Autodesk Fusion 360 part; units mm, degrees
(part 4 of 5)
  spline S251 degree 3 poles (-20.8842, 19.6004) (-20.7556, 19.6004) (-20.6902, 19.4873) (-20.7714, 19.4061) knots 0 0 0 0 1 1 1 1
  spline S252 degree 3 poles (-20.7714, 19.4061) (-20.8663, 19.3108) (-21.0022, 19.3689) (-20.9874, 19.4986) knots 0 0 0 0 1 1 1 1
  spline S253 degree 3 poles (-20.9874, 19.4986) (-20.9781, 19.577) (-20.9547, 19.6004) (-20.8842, 19.6004) knots 0 0 0 0 1 1 1 1
  spline S254 degree 3 poles (-15.859, 20.19) (-15.7052, 20.0307) (-15.4972, 19.7727) (-15.3967, 19.6166) knots 0 0 0 0 1 1 1 1
  spline S255 degree 3 poles (-15.3967, 19.6166) (-15.0184, 19.0281) (-14.932, 18.9156) (-14.7484, 18.7698) knots 0 0 0 0 1 1 1 1
  spline S256 degree 3 poles (-14.7484, 18.7698) (-14.5557, 18.6167) (-14.2304, 18.4347) (-14.1499, 18.4347) knots 0 0 0 0 1 1 1 1
  spline S257 degree 3 poles (-14.1499, 18.4347) (-14.1251, 18.4347) (-14.2407, 18.5764) (-14.4068, 18.7501) knots 0 0 0 0 1 1 1 1
  spline S258 degree 3 poles (-14.4068, 18.7501) (-14.5726, 18.9235) (-14.7934, 19.2028) (-14.8973, 19.371) knots 0 0 0 0 1 1 1 1
  spline S259 degree 3 poles (-14.8973, 19.371) (-15.2719, 19.9774) (-15.5315, 20.2477) (-15.9388, 20.4548) knots 0 0 0 0 1 1 1 1
  spline S260 degree 3 poles (-15.9388, 20.4548) (-16.2274, 20.6013) (-16.214, 20.557) (-15.859, 20.19) knots 0 0 0 0 1 1 1 1
  spline S261 degree 3 poles (-15.6155, 21.0271) (-15.2839, 20.7069) (-14.9551, 20.5714) (-14.3803, 20.5181) knots 0 0 0 0 1 1 1 1
  spline S262 degree 3 poles (-14.3803, 20.5181) (-13.7203, 20.4569) (-12.3448, 20.6853) (-12.2268, 20.8755) knots 0 0 0 0 1 1 1 1
  spline S263 degree 3 poles (-12.2268, 20.8755) (-12.2185, 20.8889) (-12.7586, 20.894) (-13.4265, 20.8875) knots 0 0 0 0 1 1 1 1
  spline S264 degree 3 poles (-13.4265, 20.8875) (-14.7814, 20.8737) (-14.9286, 20.8889) (-15.3916, 21.0928) knots 0 0 0 0 1 1 1 1
  spline S265 degree 3 poles (-15.3916, 21.0928) (-15.5622, 21.1682) (-15.7231, 21.2387) (-15.7493, 21.2504) knots 0 0 0 0 1 1 1 1
  spline S266 degree 3 poles (-15.7493, 21.2504) (-15.849, 21.2934) (-15.7905, 21.1964) (-15.6155, 21.0271) knots 0 0 0 0 1 1 1 1
  spline S267 degree 3 poles (-13.7519, -14.1202) (-12.6942, -27.0541) (-11.8189, -37.6776) (-11.8061, -37.7278) knots 0 0 0 0 1 1 1 1
  spline S268 degree 3 poles (-11.8061, -37.7278) (-11.7607, -37.9101) (-11.4151, -37.9504) (-11.326, -37.7842) knots 0 0 0 0 1 1 1 1
  spline S269 degree 3 poles (-11.326, -37.7842) (-11.2393, -37.6222) (-11.2764, 12.0151) (-11.3638, 12.1578) knots 0 0 0 0 1 1 1 1
  spline S270 degree 3 poles (-11.3638, 12.1578) (-11.5103, 12.3983) (-11.8199, 12.5135) (-12.0768, 12.4234) knots 0 0 0 0 1 1 1 1
  spline S271 degree 3 poles (-12.0768, 12.4234) (-12.3517, 12.3267) (-15.5192, 10.2626) (-15.6048, 10.1244) knots 0 0 0 0 1 1 1 1
  spline S272 degree 3 poles (-15.6048, 10.1244) (-15.7235, 9.9324) (-15.7985, 10.9155) (-13.7519, -14.1202) knots 0 0 0 0 1 1 1 1
  spline S273 degree 3 poles (-15.6055, 47.6423) (-15.59, 47.5739) (-15.5364, 47.4665) (-15.4865, 47.4036) knots 0 0 0 0 1 1 1 1
  spline S274 degree 3 poles (-15.4865, 47.4036) (-15.3713, 47.2584) (-12.158, 45.1985) (-11.9657, 45.1462) knots 0 0 0 0 1 1 1 1
  spline S275 degree 3 poles (-11.9657, 45.1462) (-11.6961, 45.0736) (-11.3941, 45.2143) (-11.273, 45.4688) knots 0 0 0 0 1 1 1 1
  spline S276 degree 3 poles (-11.273, 45.4688) (-11.2159, 45.5896) (-11.2111, 47.5797) (-11.2111, 70.4615) knots 0 0 0 0 1 1 1 1
  line L116 (-11.2111, 70.4615) -> (-11.2111, 95.3228)
  line L117 (-11.2111, 95.3228) -> (-11.3115, 95.4023)
  spline S277 degree 3 poles (-11.3115, 95.4023) (-11.4347, 95.4989) (-11.5578, 95.5031) (-11.6675, 95.4143) knots 0 0 0 0 1 1 1 1
  spline S278 degree 3 poles (-11.6675, 95.4143) (-11.748, 95.349) (-11.7989, 94.7477) (-13.6755, 71.729) knots 0 0 0 0 1 1 1 1
  spline S279 degree 3 poles (-13.6755, 71.729) (-14.7346, 58.7391) (-15.6082, 48.0334) (-15.6172, 47.9388) knots 0 0 0 0 1 1 1 1
  spline S280 degree 3 poles (-15.6172, 47.9388) (-15.6261, 47.8442) (-15.6206, 47.7108) (-15.6055, 47.6423) knots 0 0 0 0 1 1 1 1
  spline S281 degree 3 poles (-15.1442, 24.6133) (-14.6259, 24.1441) (-13.8018, 23.8731) (-13.1434, 23.9553) knots 0 0 0 0 1 1 1 1
  spline S282 degree 3 poles (-13.1434, 23.9553) (-12.8686, 23.9897) (-12.8755, 24.0144) (-13.1888, 24.1235) knots 0 0 0 0 1 1 1 1
  spline S283 degree 3 poles (-13.1888, 24.1235) (-13.4503, 24.2146) (-15.2412, 24.8506) (-15.329, 24.8836) knots 0 0 0 0 1 1 1 1
  spline S284 degree 3 poles (-15.329, 24.8836) (-15.4404, 24.9256) (-15.3609, 24.809) (-15.1442, 24.6133) knots 0 0 0 0 1 1 1 1
  spline S285 degree 3 poles (-10.2752, 18.574) (-10.171, 18.9245) (-9.569, 19.6589) (-9.3878, 19.6568) knots 0 0 0 0 1 1 1 1
  spline S286 degree 3 poles (-9.3878, 19.6568) (-9.0524, 19.6527) (-8.8275, 19.3913) (-8.8797, 19.0659) knots 0 0 0 0 1 1 1 1
  spline S287 degree 3 poles (-8.8797, 19.0659) (-8.9637, 18.5403) (-9.1202, 18.3512) (-9.5436, 18.2624) knots 0 0 0 0 1 1 1 1
  spline S288 degree 3 poles (-9.5436, 18.2624) (-9.686, 18.2325) (-9.8573, 18.1744) (-9.9243, 18.1327) knots 0 0 0 0 1 1 1 1
  spline S289 degree 3 poles (-9.9243, 18.1327) (-10.3061, 17.8968) (-10.43, 18.0523) (-10.2752, 18.574) knots 0 0 0 0 1 1 1 1
  spline S290 degree 3 poles (-4.9222, -19.0378) (-4.4427, -21.601) (-2.4986, -23.2055) (0.1206, -23.1997) knots 0 0 0 0 1 1 1 1
  spline S291 degree 3 poles (0.1206, -23.1997) (3.6706, -23.1918) (5.9848, -19.9675) (4.9739, -16.4378) knots 0 0 0 0 1 1 1 1
  spline S292 degree 3 poles (4.9739, -16.4378) (3.682, -11.9251) (-2.9984, -11.6857) (-4.6573, -16.0925) knots 0 0 0 0 1 1 1 1
  spline S293 degree 3 poles (-4.6573, -16.0925) (-4.9524, -16.8767) (-5.0738, -18.2264) (-4.9222, -19.0378) knots 0 0 0 0 1 1 1 1
  spline S294 degree 3 poles (-4.9242, 2.0967) (-4.4138, -0.7987) (-1.6762, -2.6382) (1.1996, -2.0184) knots 0 0 0 0 1 1 1 1
  spline S295 degree 3 poles (1.1996, -2.0184) (5.118, -1.174) (6.5392, 3.6521) (3.7927, 6.788) knots 0 0 0 0 1 1 1 1
  spline S296 degree 3 poles (3.7927, 6.788) (3.6317, 6.972) (3.479, 7.1223) (3.4529, 7.1223) knots 0 0 0 0 1 1 1 1
  spline S297 degree 3 poles (3.4529, 7.1223) (3.4102, 7.1223) (3.1217, 6.8375) (2.2081, 5.8937) knots 0 0 0 0 1 1 1 1
  line L118 (2.2081, 5.8937) -> (1.8882, 5.5635)
  line L119 (1.8882, 5.5635) -> (2.0781, 5.3351)
  spline S298 degree 3 poles (2.0781, 5.3351) (3.8804, 3.1695) (2.7553, 0.3099) (0.1014, 0.3099) knots 0 0 0 0 1 1 1 1
  spline S299 degree 3 poles (0.1014, 0.3099) (-2.5523, 0.3099) (-3.6774, 3.1695) (-1.8757, 5.3344) knots 0 0 0 0 1 1 1 1
  line L120 (-1.8757, 5.3344) -> (-1.6865, 5.5621)
  line L121 (-1.6865, 5.5621) -> (-1.798, 5.6828)
  spline S300 degree 3 poles (-1.798, 5.6828) (-1.8592, 5.7496) (-2.2094, 6.1197) (-2.576, 6.5056) knots 0 0 0 0 1 1 1 1
  line L122 (-2.576, 6.5056) -> (-3.2426, 7.2076)
  line L123 (-3.2426, 7.2076) -> (-3.537, 6.8939)
  spline S301 degree 3 poles (-3.537, 6.8939) (-4.1995, 6.1881) (-4.6312, 5.387) (-4.8554, 4.447) knots 0 0 0 0 1 1 1 1
  spline S302 degree 3 poles (-4.8554, 4.447) (-4.9762, 3.94) (-5.0154, 2.6123) (-4.9242, 2.0967) knots 0 0 0 0 1 1 1 1
  spline S303 degree 3 poles (-4.9222, 21.5111) (-4.4427, 18.9479) (-2.4986, 17.3434) (0.1206, 17.3492) knots 0 0 0 0 1 1 1 1
  spline S304 degree 3 poles (0.1206, 17.3492) (3.6706, 17.3571) (5.9848, 20.5814) (4.9739, 24.1111) knots 0 0 0 0 1 1 1 1
  spline S305 degree 3 poles (4.9739, 24.1111) (3.682, 28.6238) (-2.9984, 28.8629) (-4.6573, 24.4561) knots 0 0 0 0 1 1 1 1
  spline S306 degree 3 poles (-4.6573, 24.4561) (-4.9524, 23.6722) (-5.0738, 22.3225) (-4.9222, 21.5111) knots 0 0 0 0 1 1 1 1
  spline S307 degree 3 poles (-4.9222, 44.3654) (-4.4427, 41.8022) (-2.4986, 40.1973) (0.1206, 40.2032) knots 0 0 0 0 1 1 1 1
  spline S308 degree 3 poles (0.1206, 40.2032) (3.6706, 40.2111) (5.9848, 43.4354) (4.9739, 46.9654) knots 0 0 0 0 1 1 1 1
  spline S309 degree 3 poles (4.9739, 46.9654) (3.682, 51.4778) (-2.9984, 51.7172) (-4.6573, 47.3104) knots 0 0 0 0 1 1 1 1
  spline S310 degree 3 poles (-4.6573, 47.3104) (-4.9524, 46.5262) (-5.0738, 45.1765) (-4.9222, 44.3654) knots 0 0 0 0 1 1 1 1
  spline S311 degree 3 poles (-4.9222, 63.474) (-4.4427, 60.9108) (-2.4986, 59.3063) (0.1206, 59.3121) knots 0 0 0 0 1 1 1 1
  spline S312 degree 3 poles (0.1206, 59.3121) (3.6706, 59.32) (5.9848, 62.5443) (4.9739, 66.074) knots 0 0 0 0 1 1 1 1
  spline S313 degree 3 poles (4.9739, 66.074) (3.682, 70.5867) (-2.9984, 70.8258) (-4.6573, 66.419) knots 0 0 0 0 1 1 1 1
  spline S314 degree 3 poles (-4.6573, 66.419) (-4.9524, 65.6351) (-5.0738, 64.2854) (-4.9222, 63.474) knots 0 0 0 0 1 1 1 1
  spline S315 degree 3 poles (-4.9242, 84.6085) (-4.4138, 81.7131) (-1.6762, 79.8736) (1.1996, 80.4934) knots 0 0 0 0 1 1 1 1
  spline S316 degree 3 poles (1.1996, 80.4934) (5.118, 81.3378) (6.5392, 86.1639) (3.7927, 89.2998) knots 0 0 0 0 1 1 1 1
  spline S317 degree 3 poles (3.7927, 89.2998) (3.6317, 89.4835) (3.479, 89.6341) (3.4529, 89.6341) knots 0 0 0 0 1 1 1 1
  spline S318 degree 3 poles (3.4529, 89.6341) (3.4102, 89.6341) (3.1217, 89.3493) (2.2081, 88.4055) knots 0 0 0 0 1 1 1 1
  line L124 (2.2081, 88.4055) -> (1.8882, 88.0753)
  line L125 (1.8882, 88.0753) -> (2.0781, 87.8469)
  spline S319 degree 3 poles (2.0781, 87.8469) (3.8804, 85.6813) (2.7553, 82.8217) (0.1014, 82.8217) knots 0 0 0 0 1 1 1 1
  spline S320 degree 3 poles (0.1014, 82.8217) (-2.5523, 82.8217) (-3.6774, 85.6813) (-1.8757, 87.8462) knots 0 0 0 0 1 1 1 1
  line L126 (-1.8757, 87.8462) -> (-1.6865, 88.0739)
  line L127 (-1.6865, 88.0739) -> (-1.798, 88.1947)
  spline S321 degree 3 poles (-1.798, 88.1947) (-1.8592, 88.261) (-2.2094, 88.6315) (-2.576, 89.0174) knots 0 0 0 0 1 1 1 1
  line L128 (-2.576, 89.0174) -> (-3.2426, 89.7194)
  line L129 (-3.2426, 89.7194) -> (-3.537, 89.4057)
  spline S322 degree 3 poles (-3.537, 89.4057) (-4.1995, 88.6999) (-4.6312, 87.8988) (-4.8554, 86.9588) knots 0 0 0 0 1 1 1 1
  spline S323 degree 3 poles (-4.8554, 86.9588) (-4.9762, 86.4518) (-5.0154, 85.1241) (-4.9242, 84.6085) knots 0 0 0 0 1 1 1 1
  spline S324 degree 3 poles (-4.9252, 92.6341) (-4.5713, 91.0117) (-3.1164, 89.9402) (-1.5187, 90.126) knots 0 0 0 0 1 1 1 1
  spline S325 degree 3 poles (-1.5187, 90.126) (-0.1704, 90.2828) (0.499, 90.9728) (1.1549, 92.8828) knots 0 0 0 0 1 1 1 1
  spline S326 degree 3 poles (1.1549, 92.8828) (1.6144, 94.2208) (1.9742, 94.5482) (2.6239, 94.2194) knots 0 0 0 0 1 1 1 1
  spline S327 degree 3 poles (2.6239, 94.2194) (3.3851, 93.8342) (3.0343, 92.424) (2.1768, 92.424) knots 0 0 0 0 1 1 1 1
  line L130 (2.1768, 92.424) -> (2.0506, 92.424)
  line L131 (2.0506, 92.424) -> (2.0506, 91.2545)
  line L132 (2.0506, 91.2545) -> (2.0506, 90.085)
  line L133 (2.0506, 90.085) -> (2.3275, 90.1108)
  spline S328 degree 3 poles (2.3275, 90.1108) (4.2423, 90.2897) (5.3419, 91.6934) (5.1765, 93.7479) knots 0 0 0 0 1 1 1 1
  spline S329 degree 3 poles (5.1765, 93.7479) (4.9292, 96.8191) (0.8178, 97.7501) (-0.5377, 95.0418) knots 0 0 0 0 1 1 1 1
  spline S330 degree 3 poles (-0.5377, 95.0418) (-0.6794, 94.7581) (-0.8094, 94.3948) (-0.9821, 93.7998) knots 0 0 0 0 1 1 1 1
  spline S331 degree 3 poles (-0.9821, 93.7998) (-1.2934, 92.7256) (-1.4929, 92.4529) (-1.9634, 92.4563) knots 0 0 0 0 1 1 1 1
  spline S332 degree 3 poles (-1.9634, 92.4563) (-3.0624, 92.4649) (-3.1387, 94.2094) (-2.0484, 94.3911) knots 0 0 0 0 1 1 1 1
  line L134 (-2.0484, 94.3911) -> (-1.886, 94.4179)
  line L135 (-1.886, 94.4179) -> (-1.886, 95.5285)
  line L136 (-1.886, 95.5285) -> (-1.886, 96.6388)
  line L137 (-1.886, 96.6388) -> (-2.1454, 96.6147)
  spline S333 degree 3 poles (-2.1454, 96.6147) (-4.129, 96.4304) (-5.3669, 94.658) (-4.9252, 92.6341) knots 0 0 0 0 1 1 1 1
  line L138 (0.1189, -39.0827) -> (4.9168, -39.0827)
  line L139 (4.9168, -39.0827) -> (4.9161, -37.0478)
  spline S334 degree 3 poles (4.9161, -37.0478) (4.9157, -35.9282) (4.8989, -34.8097) (4.8783, -34.5617) knots 0 0 0 0 1 1 1 1
  spline S335 degree 3 poles (4.8783, -34.5617) (4.6598, -31.9245) (1.8174, -31.0416) (0.1781, -33.1012) knots 0 0 0 0 1 1 1 1
  line L140 (0.1781, -33.1012) -> (-0.017, -33.3468)
  line L141 (-0.017, -33.3468) -> (-0.3303, -33.0304)
  spline S336 degree 3 poles (-0.3303, -33.0304) (-1.5407, -31.8086) (-3.7197, -32.2936) (-4.4275, -33.9425) knots 0 0 0 0 1 1 1 1
  spline S337 degree 3 poles (-4.4275, -33.9425) (-4.6642, -34.4932) (-4.6521, -34.3474) (-4.6662, -36.8184) knots 0 0 0 0 1 1 1 1
  line L142 (-4.6662, -36.8184) -> (-4.6793, -39.0827)
  line L143 (-4.6793, -39.0827) -> (0.1189, -39.0827)
  line L144 (0.1206, -31.3629) -> (4.9168, -31.3629)
  line L145 (4.9168, -31.3629) -> (4.9168, -30.1786)
  line L146 (4.9168, -30.1786) -> (4.9168, -28.994)
  line L147 (4.9168, -28.994) -> (3.1726, -28.984)
  line L148 (3.1726, -28.984) -> (1.428, -28.9741)
  line L149 (1.428, -28.9741) -> (3.1629, -27.7854)
  line L150 (3.1629, -27.7854) -> (4.8979, -26.5963)
  line L151 (4.8979, -26.5963) -> (4.9078, -25.1197)
  spline S338 degree 3 poles (4.9078, -25.1197) (4.914, -24.1972) (4.904, -23.6427) (4.881, -23.6427) knots 0 0 0 0 1 1 1 1
  spline S339 degree 3 poles (4.881, -23.6427) (4.8611, -23.6427) (4.0655, -24.2102) (3.1131, -24.9033) knots 0 0 0 0 1 1 1 1
  spline S340 degree 3 poles (3.1131, -24.9033) (2.161, -25.5967) (1.3719, -26.1643) (1.3602, -26.1646) knots 0 0 0 0 1 1 1 1
  spline S341 degree 3 poles (1.3602, -26.1646) (1.3486, -26.165) (1.3162, -26.0762) (1.2884, -25.9675) knots 0 0 0 0 1 1 1 1
  spline S342 degree 3 poles (1.2884, -25.9675) (1.0514, -25.0433) (0.2806, -24.2983) (-0.6908, -24.0544) knots 0 0 0 0 1 1 1 1
  spline S343 degree 3 poles (-0.6908, -24.0544) (-2.3731, -23.6327) (-3.9494, -24.418) (-4.4654, -25.9352) knots 0 0 0 0 1 1 1 1
  spline S344 degree 3 poles (-4.4654, -25.9352) (-4.6683, -26.532) (-4.6759, -26.6441) (-4.6759, -29.0931) knots 0 0 0 0 1 1 1 1
  line L152 (-4.6759, -29.0931) -> (-4.6759, -31.3629)
  line L153 (-4.6759, -31.3629) -> (0.1206, -31.3629)
  line L154 (0.1206, -11.7572) -> (4.9168, -11.7572)
  line L155 (4.9168, -11.7572) -> (4.9168, -10.5726)
  line L156 (4.9168, -10.5726) -> (4.9168, -9.3881)
  line L157 (4.9168, -9.3881) -> (2.1183, -9.3784)
  line L158 (2.1183, -9.3784) -> (-0.6805, -9.3684)
  line L159 (-0.6805, -9.3684) -> (2.1183, -7.5348)
  line L160 (2.1183, -7.5348) -> (4.9168, -5.7008)
  line L161 (4.9168, -5.7008) -> (4.9168, -4.4677)
  line L162 (4.9168, -4.4677) -> (4.9168, -3.2346)
  line L163 (4.9168, -3.2346) -> (0.1206, -3.2346)
  line L164 (0.1206, -3.2346) -> (-4.6759, -3.2346)
  line L165 (-4.6759, -3.2346) -> (-4.6759, -4.4192)
  line L166 (-4.6759, -4.4192) -> (-4.6759, -5.6038)
  line L167 (-4.6759, -5.6038) -> (-1.8964, -5.6135)
  line L168 (-1.8964, -5.6135) -> (0.8832, -5.6234)
  line L169 (0.8832, -5.6234) -> (-1.8964, -7.4364)
  line L170 (-1.8964, -7.4364) -> (-4.6759, -9.2494)
  line L171 (-4.6759, -9.2494) -> (-4.6759, -10.5032)
  line L172 (-4.6759, -10.5032) -> (-4.6759, -11.7572)
  line L173 (-4.6759, -11.7572) -> (0.1206, -11.7572)
  line L174 (0.1206, 7.8102) -> (4.9168, 7.8102)
  line L175 (4.9168, 7.8102) -> (4.9168, 8.9948)
  line L176 (4.9168, 8.9948) -> (4.9168, 10.1797)
  line L177 (4.9168, 10.1797) -> (3.0061, 10.1797)
  line L178 (3.0061, 10.1797) -> (1.0951, 10.1797)
  line L179 (1.0951, 10.1797) -> (1.0951, 12.0333)
  line L180 (1.0951, 12.0333) -> (1.0951, 13.8869)
  line L181 (1.0951, 13.8869) -> (3.0061, 13.8869)
  line L182 (3.0061, 13.8869) -> (4.9168, 13.8869)
  line L183 (4.9168, 13.8869) -> (4.9168, 15.0526)
  line L184 (4.9168, 15.0526) -> (4.9168, 16.2179)
  line L185 (4.9168, 16.2179) -> (0.1206, 16.2179)
  line L186 (0.1206, 16.2179) -> (-4.6759, 16.2179)
  line L187 (-4.6759, 16.2179) -> (-4.6759, 15.0526)
  line L188 (-4.6759, 15.0526) -> (-4.6759, 13.8869)
  line L189 (-4.6759, 13.8869) -> (-2.803, 13.8869)
  line L190 (-2.803, 13.8869) -> (-0.9305, 13.8869)
  line L191 (-0.9305, 13.8869) -> (-0.9305, 12.0333)
  line L192 (-0.9305, 12.0333) -> (-0.9305, 10.1797)
  line L193 (-0.9305, 10.1797) -> (-2.803, 10.1797)
  line L194 (-2.803, 10.1797) -> (-4.6759, 10.1797)
  line L195 (-4.6759, 10.1797) -> (-4.6759, 8.9948)
  line L196 (-4.6759, 8.9948) -> (-4.6759, 7.8102)
  line L197 (-4.6759, 7.8102) -> (0.1206, 7.8102)
  line L198 (0.1206, 32.04) -> (4.9168, 32.04)
  line L199 (4.9168, 32.04) -> (4.9168, 33.2246)
  line L200 (4.9168, 33.2246) -> (4.9168, 34.4088)
  line L201 (4.9168, 34.4088) -> (3.1726, 34.4188)
  line L202 (3.1726, 34.4188) -> (1.428, 34.4288)
  line L203 (1.428, 34.4288) -> (3.1629, 35.6179)
  line L204 (3.1629, 35.6179) -> (4.8979, 36.8066)
  line L205 (4.8979, 36.8066) -> (4.9078, 38.2835)
  spline S345 degree 3 poles (4.9078, 38.2835) (4.914, 39.2057) (4.904, 39.7602) (4.881, 39.7602) knots 0 0 0 0 1 1 1 1
  spline S346 degree 3 poles (4.881, 39.7602) (4.8611, 39.7602) (4.0655, 39.193) (3.1131, 38.4995) knots 0 0 0 0 1 1 1 1
  spline S347 degree 3 poles (3.1131, 38.4995) (2.161, 37.8065) (1.3719, 37.2389) (1.3602, 37.2386) knots 0 0 0 0 1 1 1 1
  spline S348 degree 3 poles (1.3602, 37.2386) (1.3486, 37.2379) (1.3162, 37.3266) (1.2884, 37.4353) knots 0 0 0 0 1 1 1 1
  spline S349 degree 3 poles (1.2884, 37.4353) (1.0514, 38.3596) (0.2806, 39.1049) (-0.6908, 39.3484) knots 0 0 0 0 1 1 1 1
  spline S350 degree 3 poles (-0.6908, 39.3484) (-2.3731, 39.7705) (-3.9494, 38.9849) (-4.4654, 37.4677) knots 0 0 0 0 1 1 1 1
  spline S351 degree 3 poles (-4.4654, 37.4677) (-4.6683, 36.8709) (-4.6759, 36.7591) (-4.6759, 34.3098) knots 0 0 0 0 1 1 1 1
  line L206 (-4.6759, 34.3098) -> (-4.6759, 32.04)
  line L207 (-4.6759, 32.04) -> (0.1206, 32.04)
  line L208 (0.1189, 51.6456) -> (4.9168, 51.6456)
  line L209 (4.9168, 51.6456) -> (4.9161, 53.6808)
  spline S352 degree 3 poles (4.9161, 53.6808) (4.9157, 54.8001) (4.8989, 55.919) (4.8783, 56.167) knots 0 0 0 0 1 1 1 1
  spline S353 degree 3 poles (4.8783, 56.167) (4.6598, 58.8041) (1.8174, 59.687) (0.1781, 57.6271) knots 0 0 0 0 1 1 1 1
  line L210 (0.1781, 57.6271) -> (-0.017, 57.3818)
  line L211 (-0.017, 57.3818) -> (-0.3303, 57.6983)
  spline S354 degree 3 poles (-0.3303, 57.6983) (-1.5407, 58.92) (-3.7197, 58.435) (-4.4275, 56.7861) knots 0 0 0 0 1 1 1 1
  spline S355 degree 3 poles (-4.4275, 56.7861) (-4.6642, 56.2354) (-4.6521, 56.3809) (-4.6662, 53.9103) knots 0 0 0 0 1 1 1 1
  line L212 (-4.6662, 53.9103) -> (-4.6793, 51.6456)
  line L213 (-4.6793, 51.6456) -> (0.1189, 51.6456)
  line L214 (-3.644, 69.6464) -> (-2.6121, 69.6464)
  line L215 (-2.6121, 69.6464) -> (-2.6121, 70.7164)
  line L216 (-2.6121, 70.7164) -> (-2.6121, 71.7865)
  line L217 (-2.6121, 71.7865) -> (1.1525, 71.7865)
  line L218 (1.1525, 71.7865) -> (4.9168, 71.7865)
  line L219 (4.9168, 71.7865) -> (4.9168, 72.9711)
  line L220 (4.9168, 72.9711) -> (4.9168, 74.156)
  line L221 (4.9168, 74.156) -> (1.1525, 74.156)
  line L222 (1.1525, 74.156) -> (-2.6121, 74.156)
  line L223 (-2.6121, 74.156) -> (-2.6121, 75.2453)
  line L224 (-2.6121, 75.2453) -> (-2.6121, 76.3343)
  line L225 (-2.6121, 76.3343) -> (-3.644, 76.3343)
  line L226 (-3.644, 76.3343) -> (-4.6759, 76.3343)
  line L227 (-4.6759, 76.3343) -> (-4.6759, 72.9903)
  line L228 (-4.6759, 72.9903) -> (-4.6759, 69.6464)
  line L229 (-4.6759, 69.6464) -> (-3.644, 69.6464)
  line L230 (0.1206, 76.9458) -> (4.9168, 76.9458)
  line L231 (4.9168, 76.9458) -> (4.9168, 78.1304)
  line L232 (4.9168, 78.1304) -> (4.9168, 79.3154)
  line L233 (4.9168, 79.3154) -> (0.1206, 79.3154)
  line L234 (0.1206, 79.3154) -> (-4.6759, 79.3154)
  line L235 (-4.6759, 79.3154) -> (-4.6759, 78.1304)
  line L236 (-4.6759, 78.1304) -> (-4.6759, 76.9458)
  line L237 (-4.6759, 76.9458) -> (0.1206, 76.9458)
  spline S356 degree 3 poles (-4.4272, -17.1529) (-3.5357, -12.5222) (3.3672, -12.2945) (4.5343, -16.8571) knots 0 0 0 0 1 1 1 1
  spline S357 degree 3 poles (4.5343, -16.8571) (5.2993, -19.8489) (3.1846, -22.5778) (0.1014, -22.5778) knots 0 0 0 0 1 1 1 1
  spline S358 degree 3 poles (0.1014, -22.5778) (-2.8794, -22.5778) (-4.9861, -20.0545) (-4.4272, -17.1529) knots 0 0 0 0 1 1 1 1
  spline S359 degree 3 poles (-4.4833, 3.68) (-4.3832, 4.6551) (-4.012, 5.5528) (-3.45, 6.1795) knots 0 0 0 0 1 1 1 1
  line L238 (-3.45, 6.1795) -> (-3.2502, 6.4024)
  line L239 (-3.2502, 6.4024) -> (-2.8202, 5.9738)
  line L240 (-2.8202, 5.9738) -> (-2.3903, 5.5449)
  line L241 (-2.3903, 5.5449) -> (-2.5193, 5.3654)
  spline S360 degree 3 poles (-2.5193, 5.3654) (-3.4844, 4.0219) (-3.4603, 1.9746) (-2.4656, 0.7924) knots 0 0 0 0 1 1 1 1
  spline S361 degree 3 poles (-2.4656, 0.7924) (-1.1933, -0.7193) (1.396, -0.7193) (2.6683, 0.7924) knots 0 0 0 0 1 1 1 1
  spline S362 degree 3 poles (2.6683, 0.7924) (3.6589, 1.9695) (3.6913, 4.0449) (2.7385, 5.3107) knots 0 0 0 0 1 1 1 1
  line L242 (2.7385, 5.3107) -> (2.592, 5.5057)
  line L243 (2.592, 5.5057) -> (3.0309, 5.9411)
  line L244 (3.0309, 5.9411) -> (3.4697, 6.3769)
  line L245 (3.4697, 6.3769) -> (3.6053, 6.2242)
  spline S363 degree 3 poles (3.6053, 6.2242) (5.6553, 3.9073) (4.7868, 0.0484) (1.9491, -1.1327) knots 0 0 0 0 1 1 1 1
  spline S364 degree 3 poles (1.9491, -1.1327) (-1.4014, -2.5275) (-4.8551, 0.0564) (-4.4833, 3.68) knots 0 0 0 0 1 1 1 1
  spline S365 degree 3 poles (-4.4272, 23.396) (-3.5357, 28.0267) (3.3672, 28.2544) (4.5343, 23.6918) knots 0 0 0 0 1 1 1 1
  spline S366 degree 3 poles (4.5343, 23.6918) (5.2993, 20.7) (3.1846, 17.9711) (0.1014, 17.9711) knots 0 0 0 0 1 1 1 1
  spline S367 degree 3 poles (0.1014, 17.9711) (-2.8794, 17.9711) (-4.9861, 20.4944) (-4.4272, 23.396) knots 0 0 0 0 1 1 1 1
  spline S368 degree 3 poles (-4.4272, 46.25) (-3.5357, 50.8807) (3.3672, 51.1084) (4.5343, 46.5458) knots 0 0 0 0 1 1 1 1
  spline S369 degree 3 poles (4.5343, 46.5458) (5.2993, 43.5544) (3.1846, 40.825) (0.1014, 40.825) knots 0 0 0 0 1 1 1 1
  spline S370 degree 3 poles (0.1014, 40.825) (-2.8794, 40.825) (-4.9861, 43.3483) (-4.4272, 46.25) knots 0 0 0 0 1 1 1 1
  spline S371 degree 3 poles (-4.4272, 65.3589) (-3.5357, 69.9896) (3.3672, 70.2173) (4.5343, 65.6547) knots 0 0 0 0 1 1 1 1
  spline S372 degree 3 poles (4.5343, 65.6547) (5.2993, 62.663) (3.1846, 59.934) (0.1014, 59.934) knots 0 0 0 0 1 1 1 1
  spline S373 degree 3 poles (0.1014, 59.934) (-2.8794, 59.934) (-4.9861, 62.4573) (-4.4272, 65.3589) knots 0 0 0 0 1 1 1 1
  spline S374 degree 3 poles (-4.4833, 86.1914) (-4.3832, 87.1669) (-4.012, 88.0646) (-3.45, 88.6913) knots 0 0 0 0 1 1 1 1
  line L246 (-3.45, 88.6913) -> (-3.2502, 88.9142)
  line L247 (-3.2502, 88.9142) -> (-2.8202, 88.4856)
  line L248 (-2.8202, 88.4856) -> (-2.3903, 88.0567)
  line L249 (-2.3903, 88.0567) -> (-2.5193, 87.8772)
  spline S375 degree 3 poles (-2.5193, 87.8772) (-3.4844, 86.5337) (-3.4603, 84.4864) (-2.4656, 83.3042) knots 0 0 0 0 1 1 1 1
  spline S376 degree 3 poles (-2.4656, 83.3042) (-1.1933, 81.7926) (1.396, 81.7926) (2.6683, 83.3042) knots 0 0 0 0 1 1 1 1
  spline S377 degree 3 poles (2.6683, 83.3042) (3.6589, 84.4813) (3.6913, 86.5567) (2.7385, 87.8225) knots 0 0 0 0 1 1 1 1
  line L250 (2.7385, 87.8225) -> (2.592, 88.0175)
  line L251 (2.592, 88.0175) -> (3.0309, 88.453)
  line L252 (3.0309, 88.453) -> (3.4697, 88.8887)
  line L253 (3.4697, 88.8887) -> (3.6053, 88.736)
  spline S378 degree 3 poles (3.6053, 88.736) (5.6553, 86.4188) (4.7868, 82.5603) (1.9491, 81.3791) knots 0 0 0 0 1 1 1 1
  spline S379 degree 3 poles (1.9491, 81.3791) (-1.4014, 79.9844) (-4.8551, 82.5682) (-4.4833, 86.1914) knots 0 0 0 0 1 1 1 1
  spline S380 degree 3 poles (-4.4062, 94.2201) (-4.1665, 95.0831) (-3.5161, 95.7459) (-2.7019, 95.9557) knots 0 0 0 0 1 1 1 1
  spline S381 degree 3 poles (-2.7019, 95.9557) (-2.3167, 96.0551) (-2.3445, 96.0943) (-2.3445, 95.4529) knots 0 0 0 0 1 1 1 1
  line L254 (-2.3445, 95.4529) -> (-2.3445, 94.8891)
  line L255 (-2.3445, 94.8891) -> (-2.5557, 94.7787)
  spline S382 degree 3 poles (-2.5557, 94.7787) (-3.0576, 94.5166) (-3.3, 94.0681) (-3.3, 93.4015) knots 0 0 0 0 1 1 1 1
  spline S383 degree 3 poles (-3.3, 93.4015) (-3.3, 92.4412) (-2.8226, 91.908) (-1.9624, 91.908) knots 0 0 0 0 1 1 1 1
  spline S384 degree 3 poles (-1.9624, 91.908) (-1.1761, 91.908) (-0.9512, 92.1687) (-0.5112, 93.5886) knots 0 0 0 0 1 1 1 1
  spline S385 degree 3 poles (-0.5112, 93.5886) (-0.0166, 95.1856) (0.4175, 95.7315) (1.3909, 95.9805) knots 0 0 0 0 1 1 1 1
  spline S386 degree 3 poles (1.3909, 95.9805) (2.6191, 96.2945) (3.8983, 95.6933) (4.4435, 94.5451) knots 0 0 0 0 1 1 1 1
  spline S387 degree 3 poles (4.4435, 94.5451) (5.1954, 92.9619) (4.2701, 90.9281) (2.7034, 90.72) knots 0 0 0 0 1 1 1 1
  line L256 (2.7034, 90.72) -> (2.5091, 90.6942)
  line L257 (2.5091, 90.6942) -> (2.5091, 91.2865)
  line L258 (2.5091, 91.2865) -> (2.5091, 91.8788)
  line L259 (2.5091, 91.8788) -> (2.6989, 91.9576)
  spline S388 degree 3 poles (2.6989, 91.9576) (4.0459, 92.5172) (3.727, 94.8086) (2.2951, 94.8637) knots 0 0 0 0 1 1 1 1
  spline S389 degree 3 poles (2.2951, 94.8637) (1.5157, 94.8932) (1.2123, 94.5692) (0.7146, 93.1738) knots 0 0 0 0 1 1 1 1
  spline S390 degree 3 poles (0.7146, 93.1738) (0.0811, 91.3983) (-0.4552, 90.8228) (-1.584, 90.7059) knots 0 0 0 0 1 1 1 1
  spline S391 degree 3 poles (-1.584, 90.7059) (-3.4789, 90.5095) (-4.9335, 92.3211) (-4.4062, 94.2201) knots 0 0 0 0 1 1 1 1
  spline S392 degree 3 poles (-4.0905, -34.5173) (-3.4607, -32.7349) (-1.1661, -32.414) (-0.1848, -33.9711) knots 0 0 0 0 1 1 1 1
  spline S393 degree 3 poles (-0.1848, -33.9711) (-0.0314, -34.2143) (0.0487, -34.2105) (0.2042, -33.9522) knots 0 0 0 0 1 1 1 1
  spline S394 degree 3 poles (0.2042, -33.9522) (1.3324, -32.0776) (3.748, -32.2062) (4.3283, -34.172) knots 0 0 0 0 1 1 1 1
  spline S395 degree 3 poles (4.3283, -34.172) (4.3881, -34.3756) (4.3974, -34.6277) (4.4101, -36.4362) knots 0 0 0 0 1 1 1 1
  line L260 (4.4101, -36.4362) -> (4.4242, -38.4714)
  line L261 (4.4242, -38.4714) -> (0.1017, -38.4714)
  line L262 (0.1017, -38.4714) -> (-4.2212, -38.4714)
  line L263 (-4.2212, -38.4714) -> (-4.2095, -36.6464)
  line L264 (-4.2095, -36.6464) -> (-4.1981, -34.8214)
  line L265 (-4.1981, -34.8214) -> (-4.0905, -34.5173)
  spline S396 degree 3 poles (-4.1242, -26.5856) (-3.7685, -25.3064) (-2.8202, -24.5852) (-1.5036, -24.5924) knots 0 0 0 0 1 1 1 1
  spline S397 degree 3 poles (-1.5036, -24.5924) (-0.1456, -24.5996) (0.6599, -25.2951) (0.9275, -26.6916) knots 0 0 0 0 1 1 1 1
  spline S398 degree 3 poles (0.9275, -26.6916) (0.9891, -27.0118) (1.0032, -27.0441) (1.0813, -27.0441) knots 0 0 0 0 1 1 1 1
  spline S399 degree 3 poles (1.0813, -27.0441) (1.1336, -27.0441) (1.7947, -26.588) (2.7698, -25.8784) knots 0 0 0 0 1 1 1 1
  spline S400 degree 3 poles (2.7698, -25.8784) (3.651, -25.2377) (4.383, -24.7131) (4.396, -24.7131) knots 0 0 0 0 1 1 1 1
  spline S401 degree 3 poles (4.396, -24.7131) (4.4094, -24.7131) (4.4201, -25.045) (4.4201, -25.4506) knots 0 0 0 0 1 1 1 1
  line L266 (4.4201, -25.4506) -> (4.4201, -26.1884)
  line L267 (4.4201, -26.1884) -> (2.7203, -27.352)
  line L268 (2.7203, -27.352) -> (1.0204, -28.5156)
  line L269 (1.0204, -28.5156) -> (1.0194, -29.0601)
  line L270 (1.0194, -29.0601) -> (1.0187, -29.6049)
  line L271 (1.0187, -29.6049) -> (2.7192, -29.6049)
  line L272 (2.7192, -29.6049) -> (4.4201, -29.6049)
  line L273 (4.4201, -29.6049) -> (4.4201, -30.1779)
  line L274 (4.4201, -30.1779) -> (4.4201, -30.7513)
  line L275 (4.4201, -30.7513) -> (0.0989, -30.7513)
  line L276 (0.0989, -30.7513) -> (-4.2222, -30.7513)
  line L277 (-4.2222, -30.7513) -> (-4.2078, -28.7928)
  spline S402 degree 3 poles (-4.2078, -28.7928) (-4.1947, -27.05) (-4.1854, -26.8068) (-4.1242, -26.5856) knots 0 0 0 0 1 1 1 1
  line L278 (-0.8937, -7.4939) -> (2.4296, -5.3176)
  line L279 (2.4296, -5.3176) -> (2.4313, -5.155)
  line L280 (2.4313, -5.155) -> (2.4327, -4.9926)
  line L281 (2.4327, -4.9926) -> (-0.8923, -4.9926)
  line L282 (-0.8923, -4.9926) -> (-4.217, -4.9926)
  line L283 (-4.217, -4.9926) -> (-4.217, -4.4196)
  line L284 (-4.217, -4.4196) -> (-4.217, -3.8462)
  line L285 (-4.217, -3.8462) -> (0.1014, -3.8462)
  line L286 (0.1014, -3.8462) -> (4.4201, -3.8462)
  line L287 (4.4201, -3.8462) -> (4.4177, -4.5819)
  line L288 (4.4177, -4.5819) -> (4.4156, -5.3176)
  line L289 (4.4156, -5.3176) -> (1.0641, -7.5169)
  line L290 (1.0641, -7.5169) -> (-2.2871, -9.7162)
  line L291 (-2.2871, -9.7162) -> (-2.2991, -9.8576)
  line L292 (-2.2991, -9.8576) -> (-2.3108, -9.9993)
  line L293 (-2.3108, -9.9993) -> (1.0545, -9.9993)
  line L294 (1.0545, -9.9993) -> (4.4201, -9.9993)
  line L295 (4.4201, -9.9993) -> (4.4201, -10.5723)
  line L296 (4.4201, -10.5723) -> (4.4201, -11.1457)
  line L297 (4.4201, -11.1457) -> (0.1014, -11.1457)
  line L298 (0.1014, -11.1457) -> (-4.217, -11.1457)
  line L299 (-4.217, -11.1457) -> (-4.217, -10.4079)
  line L300 (-4.217, -10.4079) -> (-4.217, -9.6701)
  line L301 (-4.217, -9.6701) -> (-0.8937, -7.4939)
  line L302 (-2.3445, 9.5682) -> (-0.4717, 9.5682)
  line L303 (-0.4717, 9.5682) -> (-0.4717, 12.0333)
  line L304 (-0.4717, 12.0333) -> (-0.4717, 14.4981)
  line L305 (-0.4717, 14.4981) -> (-2.3445, 14.4981)
  line L306 (-2.3445, 14.4981) -> (-4.217, 14.4981)
  line L307 (-4.217, 14.4981) -> (-4.217, 15.0526)
  line L308 (-4.217, 15.0526) -> (-4.217, 15.6067)
  line L309 (-4.217, 15.6067) -> (0.1014, 15.6067)
  line L310 (0.1014, 15.6067) -> (4.4201, 15.6067)
  line L311 (4.4201, 15.6067) -> (4.4201, 15.0526)
  line L312 (4.4201, 15.0526) -> (4.4201, 14.4981)
  line L313 (4.4201, 14.4981) -> (2.5283, 14.4981)
  line L314 (2.5283, 14.4981) -> (0.6366, 14.4981)
  line L315 (0.6366, 14.4981) -> (0.6366, 12.0333)
  line L316 (0.6366, 12.0333) -> (0.6366, 9.5682)
  line L317 (0.6366, 9.5682) -> (2.5283, 9.5682)
  line L318 (2.5283, 9.5682) -> (4.4201, 9.5682)
  line L319 (4.4201, 9.5682) -> (4.4201, 8.9948)
  line L320 (4.4201, 8.9948) -> (4.4201, 8.4218)
  line L321 (4.4201, 8.4218) -> (0.1014, 8.4218)
  line L322 (0.1014, 8.4218) -> (-4.217, 8.4218)
  line L323 (-4.217, 8.4218) -> (-4.217, 8.9948)
  line L324 (-4.217, 8.9948) -> (-4.217, 9.5682)
  line L325 (-4.217, 9.5682) -> (-2.3445, 9.5682)
  spline S403 degree 3 poles (-4.1242, 36.8172) (-3.7685, 38.0964) (-2.8202, 38.818) (-1.5036, 38.8108) knots 0 0 0 0 1 1 1 1
  spline S404 degree 3 poles (-1.5036, 38.8108) (-0.1456, 38.8033) (0.6599, 38.1078) (0.9275, 36.7113) knots 0 0 0 0 1 1 1 1
  spline S405 degree 3 poles (0.9275, 36.7113) (0.9891, 36.3911) (1.0032, 36.3588) (1.0813, 36.3588) knots 0 0 0 0 1 1 1 1
  spline S406 degree 3 poles (1.0813, 36.3588) (1.1336, 36.3588) (1.7947, 36.8152) (2.7698, 37.5244) knots 0 0 0 0 1 1 1 1
  spline S407 degree 3 poles (2.7698, 37.5244) (3.651, 38.1656) (4.383, 38.6901) (4.396, 38.6901) knots 0 0 0 0 1 1 1 1
  spline S408 degree 3 poles (4.396, 38.6901) (4.4094, 38.6901) (4.4201, 38.3582) (4.4201, 37.9523) knots 0 0 0 0 1 1 1 1
  line L326 (4.4201, 37.9523) -> (4.4201, 37.2149)
  line L327 (4.4201, 37.2149) -> (2.7203, 36.0509)
  line L328 (2.7203, 36.0509) -> (1.0204, 34.8873)
  line L329 (1.0204, 34.8873) -> (1.0194, 34.3428)
  line L330 (1.0194, 34.3428) -> (1.0187, 33.7983)
  line L331 (1.0187, 33.7983) -> (2.7192, 33.7983)
  line L332 (2.7192, 33.7983) -> (4.4201, 33.7983)
  line L333 (4.4201, 33.7983) -> (4.4201, 33.2249)
  line L334 (4.4201, 33.2249) -> (4.4201, 32.6516)
  line L335 (4.4201, 32.6516) -> (0.0989, 32.6516)
  line L336 (0.0989, 32.6516) -> (-4.2222, 32.6516)
  line L337 (-4.2222, 32.6516) -> (-4.2078, 34.6104)
  spline S409 degree 3 poles (-4.2078, 34.6104) (-4.1947, 36.3529) (-4.1854, 36.5964) (-4.1242, 36.8172) knots 0 0 0 0 1 1 1 1
  spline S410 degree 3 poles (-4.0905, 56.2113) (-3.4607, 57.9937) (-1.1661, 58.3146) (-0.1848, 56.7575) knots 0 0 0 0 1 1 1 1
  spline S411 degree 3 poles (-0.1848, 56.7575) (-0.0314, 56.514) (0.0487, 56.5181) (0.2042, 56.7765) knots 0 0 0 0 1 1 1 1
  spline S412 degree 3 poles (0.2042, 56.7765) (1.3324, 58.651) (3.748, 58.5224) (4.3283, 56.5567) knots 0 0 0 0 1 1 1 1
  spline S413 degree 3 poles (4.3283, 56.5567) (4.3881, 56.353) (4.3974, 56.1009) (4.4101, 54.2924) knots 0 0 0 0 1 1 1 1
  line L338 (4.4101, 54.2924) -> (4.4242, 52.2572)
  line L339 (4.4242, 52.2572) -> (0.1017, 52.2572)
  line L340 (0.1017, 52.2572) -> (-4.2212, 52.2572)
  line L341 (-4.2212, 52.2572) -> (-4.2095, 54.0822)
  line L342 (-4.2095, 54.0822) -> (-4.1981, 55.9069)
  line L343 (-4.1981, 55.9069) -> (-4.0905, 56.2113)
  line L344 (-3.644, 75.7227) -> (-3.0706, 75.7227)
  line L345 (-3.0706, 75.7227) -> (-3.0706, 74.6338)
  line L346 (-3.0706, 74.6338) -> (-3.0706, 73.5444)
  line L347 (-3.0706, 73.5444) -> (0.6747, 73.5444)
  line L348 (0.6747, 73.5444) -> (4.4201, 73.5444)
  line L349 (4.4201, 73.5444) -> (4.4201, 72.9711)
  line L350 (4.4201, 72.9711) -> (4.4201, 72.398)
  line L351 (4.4201, 72.398) -> (0.6747, 72.398)
  line L352 (0.6747, 72.398) -> (-3.0706, 72.398)
  line L353 (-3.0706, 72.398) -> (-3.0706, 71.328)
  line L354 (-3.0706, 71.328) -> (-3.0706, 70.2579)
  line L355 (-3.0706, 70.2579) -> (-3.644, 70.2579)
  line L356 (-3.644, 70.2579) -> (-4.217, 70.2579)
  line L357 (-4.217, 70.2579) -> (-4.217, 72.9903)
  line L358 (-4.217, 72.9903) -> (-4.217, 75.7227)
  line L359 (-4.217, 75.7227) -> (-3.644, 75.7227)
  line L360 (0.1014, 78.7038) -> (4.4201, 78.7038)
  line L361 (4.4201, 78.7038) -> (4.4201, 78.1304)
  line L362 (4.4201, 78.1304) -> (4.4201, 77.5574)
  line L363 (4.4201, 77.5574) -> (0.1014, 77.5574)
  line L364 (0.1014, 77.5574) -> (-4.217, 77.5574)
  line L365 (-4.217, 77.5574) -> (-4.217, 78.1304)
  line L366 (-4.217, 78.1304) -> (-4.217, 78.7038)
  line L367 (-4.217, 78.7038) -> (0.1014, 78.7038)
  spline S414 degree 3 poles (-3.1601, -18.8841) (-2.8178, -20.4814) (-1.6085, -21.4108) (0.1206, -21.4046) knots 0 0 0 0 1 1 1 1
  spline S415 degree 3 poles (0.1206, -21.4046) (2.409, -21.3967) (3.8753, -19.551) (3.4044, -17.2709) knots 0 0 0 0 1 1 1 1
  spline S416 degree 3 poles (3.4044, -17.2709) (2.7285, -13.9992) (-2.0525, -13.7092) (-3.0637, -16.8784) knots 0 0 0 0 1 1 1 1
  spline S417 degree 3 poles (-3.0637, -16.8784) (-3.2347, -17.4136) (-3.2787, -18.3306) (-3.1601, -18.8841) knots 0 0 0 0 1 1 1 1
  spline S418 degree 3 poles (-3.1601, 21.6648) (-2.8178, 20.0675) (-1.6085, 19.1381) (0.1206, 19.144) knots 0 0 0 0 1 1 1 1
  spline S419 degree 3 poles (0.1206, 19.144) (2.409, 19.1522) (3.8753, 20.9979) (3.4044, 23.278) knots 0 0 0 0 1 1 1 1
  spline S420 degree 3 poles (3.4044, 23.278) (2.7285, 26.5497) (-2.0525, 26.8397) (-3.0637, 23.6705) knots 0 0 0 0 1 1 1 1
  spline S421 degree 3 poles (-3.0637, 23.6705) (-3.2347, 23.1349) (-3.2787, 22.2183) (-3.1601, 21.6648) knots 0 0 0 0 1 1 1 1
  spline S422 degree 3 poles (-3.1601, 44.5188) (-2.8178, 42.9215) (-1.6085, 41.9921) (0.1206, 41.9983) knots 0 0 0 0 1 1 1 1
  spline S423 degree 3 poles (0.1206, 41.9983) (2.409, 42.0062) (3.8753, 43.8522) (3.4044, 46.132) knots 0 0 0 0 1 1 1 1
  spline S424 degree 3 poles (3.4044, 46.132) (2.7285, 49.4037) (-2.0525, 49.694) (-3.0637, 46.5248) knots 0 0 0 0 1 1 1 1
  spline S425 degree 3 poles (-3.0637, 46.5248) (-3.2347, 45.9892) (-3.2787, 45.0726) (-3.1601, 44.5188) knots 0 0 0 0 1 1 1 1
  spline S426 degree 3 poles (-3.1601, 63.6278) (-2.8178, 62.0304) (-1.6085, 61.101) (0.1206, 61.1069) knots 0 0 0 0 1 1 1 1
  spline S427 degree 3 poles (0.1206, 61.1069) (2.409, 61.1152) (3.8753, 62.9608) (3.4044, 65.2409) knots 0 0 0 0 1 1 1 1
  spline S428 degree 3 poles (3.4044, 65.2409) (2.7285, 68.5127) (-2.0525, 68.8026) (-3.0637, 65.6334) knots 0 0 0 0 1 1 1 1
  spline S429 degree 3 poles (-3.0637, 65.6334) (-3.2347, 65.0978) (-3.2787, 64.1812) (-3.1601, 63.6278) knots 0 0 0 0 1 1 1 1
  line L368 (-1.6188, -29.6049) -> (-0.0861, -29.6049)
  line L369 (-0.0861, -29.6049) -> (-0.0975, -28.1431)
  line L370 (-0.0975, -28.1431) -> (-0.1088, -26.6812)
  line L371 (-0.1088, -26.6812) -> (-0.2137, -26.4821)
  spline S430 degree 3 poles (-0.2137, -26.4821) (-0.7998, -25.3704) (-2.4522, -25.3835) (-3.0042, -26.5041) knots 0 0 0 0 1 1 1 1
  line L372 (-3.0042, -26.5041) -> (-3.1281, -26.7559)
  line L373 (-3.1281, -26.7559) -> (-3.1398, -28.1802)
  line L374 (-3.1398, -28.1802) -> (-3.1515, -29.6049)
  line L375 (-3.1515, -29.6049) -> (-1.6188, -29.6049)
  line L376 (-1.6188, 33.7983) -> (-0.0861, 33.7983)
  line L377 (-0.0861, 33.7983) -> (-0.0975, 35.2601)
  line L378 (-0.0975, 35.2601) -> (-0.1088, 36.722)
  line L379 (-0.1088, 36.722) -> (-0.2137, 36.9211)
  spline S431 degree 3 poles (-0.2137, 36.9211) (-0.7998, 38.0328) (-2.4522, 38.0194) (-3.0042, 36.8988) knots 0 0 0 0 1 1 1 1
  line L380 (-3.0042, 36.8988) -> (-3.1281, 36.6473)
  line L381 (-3.1281, 36.6473) -> (-3.1398, 35.2227)
  line L382 (-3.1398, 35.2227) -> (-3.1515, 33.7983)
  line L383 (-3.1515, 33.7983) -> (-1.6188, 33.7983)
  line L384 (-1.7691, -37.3629) -> (-0.4294, -37.3629)
  line L385 (-0.4294, -37.3629) -> (-0.4411, -36.245)
  line L386 (-0.4411, -36.245) -> (-0.4528, -35.1271)
  line L387 (-0.4528, -35.1271) -> (-0.5542, -34.9104)
  spline S432 degree 3 poles (-0.5542, -34.9104) (-1.0344, -33.8865) (-2.4319, -33.8456) (-2.9382, -34.8406) knots 0 0 0 0 1 1 1 1
  spline S433 degree 3 poles (-2.9382, -34.8406) (-3.0864, -35.132) (-3.1078, -35.3249) (-3.1085, -36.3599) knots 0 0 0 0 1 1 1 1
  line L388 (-3.1085, -36.3599) -> (-3.1088, -37.3629)
  line L389 (-3.1088, -37.3629) -> (-1.7691, -37.3629)
  line L390 (-1.7691, 53.3654) -> (-0.4294, 53.3654)
  line L391 (-0.4294, 53.3654) -> (-0.4411, 54.4833)
  line L392 (-0.4411, 54.4833) -> (-0.4528, 55.6012)
  line L393 (-0.4528, 55.6012) -> (-0.5542, 55.8182)
  spline S434 degree 3 poles (-0.5542, 55.8182) (-1.0344, 56.8422) (-2.4319, 56.8827) (-2.9382, 55.888) knots 0 0 0 0 1 1 1 1
  spline S435 degree 3 poles (-2.9382, 55.888) (-3.0864, 55.5967) (-3.1078, 55.4037) (-3.1085, 54.3687) knots 0 0 0 0 1 1 1 1
  line L394 (-3.1085, 54.3687) -> (-3.1088, 53.3654)
  line L395 (-3.1088, 53.3654) -> (-1.7691, 53.3654)
  spline S436 degree 3 poles (-2.6479, -17.2613) (-1.9445, -14.7259) (1.955, -14.619) (2.7918, -17.1116) knots 0 0 0 0 1 1 1 1
  spline S437 degree 3 poles (2.7918, -17.1116) (3.4343, -19.0251) (2.1135, -20.8051) (0.0632, -20.7896) knots 0 0 0 0 1 1 1 1
  spline S438 degree 3 poles (0.0632, -20.7896) (-1.8884, -20.7748) (-3.1628, -19.1162) (-2.6479, -17.2613) knots 0 0 0 0 1 1 1 1
  spline S439 degree 3 poles (-2.6479, 23.2876) (-1.9445, 25.8226) (1.955, 25.9299) (2.7918, 23.4373) knots 0 0 0 0 1 1 1 1
  spline S440 degree 3 poles (2.7918, 23.4373) (3.4343, 21.5238) (2.1135, 19.7435) (0.0632, 19.7593) knots 0 0 0 0 1 1 1 1
  spline S441 degree 3 poles (0.0632, 19.7593) (-1.8884, 19.7741) (-3.1628, 21.4327) (-2.6479, 23.2876) knots 0 0 0 0 1 1 1 1
  spline S442 degree 3 poles (-2.6479, 46.142) (-1.9445, 48.6769) (1.955, 48.7842) (2.7918, 46.2916) knots 0 0 0 0 1 1 1 1
  spline S443 degree 3 poles (2.7918, 46.2916) (3.4343, 44.3781) (2.1135, 42.5978) (0.0632, 42.6133) knots 0 0 0 0 1 1 1 1
  spline S444 degree 3 poles (0.0632, 42.6133) (-1.8884, 42.6281) (-3.1628, 44.2866) (-2.6479, 46.142) knots 0 0 0 0 1 1 1 1
  spline S445 degree 3 poles (-2.6479, 65.2506) (-1.9445, 67.7855) (1.955, 67.8928) (2.7918, 65.4002) knots 0 0 0 0 1 1 1 1
  spline S446 degree 3 poles (2.7918, 65.4002) (3.4343, 63.4867) (2.1135, 61.7064) (0.0632, 61.7222) knots 0 0 0 0 1 1 1 1
  spline S447 degree 3 poles (0.0632, 61.7222) (-1.8884, 61.737) (-3.1628, 63.3956) (-2.6479, 65.2506) knots 0 0 0 0 1 1 1 1
  spline S448 degree 3 poles (-2.6379, -27.0187) (-2.4398, -26.2558) (-1.3433, -26.0339) (-0.7812, -26.6434) knots 0 0 0 0 1 1 1 1
  spline S449 degree 3 poles (-0.7812, -26.6434) (-0.5659, -26.8773) (-0.5487, -26.9801) (-0.5484, -28.0474) knots 0 0 0 0 1 1 1 1
  line L396 (-0.5484, -28.0474) -> (-0.5484, -28.9933)
  line L397 (-0.5484, -28.9933) -> (-1.6184, -28.9933)
  line L398 (-1.6184, -28.9933) -> (-2.6885, -28.9933)
  line L399 (-2.6885, -28.9933) -> (-2.6885, -28.1035)
  spline S450 degree 3 poles (-2.6885, -28.1035) (-2.6885, -27.4892) (-2.6727, -27.1535) (-2.6379, -27.0187) knots 0 0 0 0 1 1 1 1
  spline S451 degree 3 poles (-2.6379, 36.3842) (-2.4398, 37.1474) (-1.3433, 37.3693) (-0.7812, 36.7598) knots 0 0 0 0 1 1 1 1
  spline S452 degree 3 poles (-0.7812, 36.7598) (-0.5659, 36.5259) (-0.5487, 36.4231) (-0.5484, 35.3554) knots 0 0 0 0 1 1 1 1
  line L400 (-0.5484, 35.3554) -> (-0.5484, 34.4095)
  line L401 (-0.5484, 34.4095) -> (-1.6184, 34.4095)
  line L402 (-1.6184, 34.4095) -> (-2.6885, 34.4095)
  line L403 (-2.6885, 34.4095) -> (-2.6885, 35.2994)
  spline S453 degree 3 poles (-2.6885, 35.2994) (-2.6885, 35.9137) (-2.6727, 36.2497) (-2.6379, 36.3842) knots 0 0 0 0 1 1 1 1
  spline S454 degree 3 poles (-2.5595, -35.2802) (-2.3057, -34.6948) (-1.5483, -34.5713) (-1.1149, -35.0449) knots 0 0 0 0 1 1 1 1
  spline S455 degree 3 poles (-1.1149, -35.0449) (-0.9381, -35.2382) (-0.8923, -35.4646) (-0.8923, -36.147) knots 0 0 0 0 1 1 1 1
  line L404 (-0.8923, -36.147) -> (-0.8923, -36.7517)
  line L405 (-0.8923, -36.7517) -> (-1.7756, -36.7517)
  line L406 (-1.7756, -36.7517) -> (-2.6589, -36.7517)
  line L407 (-2.6589, -36.7517) -> (-2.6424, -36.0923)
  spline S456 degree 3 poles (-2.6424, -36.0923) (-2.6297, -35.5781) (-2.6114, -35.3992) (-2.5595, -35.2802) knots 0 0 0 0 1 1 1 1
  spline S457 degree 3 poles (-2.5595, 55.4484) (-2.3057, 56.0339) (-1.5483, 56.157) (-1.1149, 55.6837) knots 0 0 0 0 1 1 1 1
  spline S458 degree 3 poles (-1.1149, 55.6837) (-0.9381, 55.4904) (-0.8923, 55.2641) (-0.8923, 54.5817) knots 0 0 0 0 1 1 1 1
  line L408 (-0.8923, 54.5817) -> (-0.8923, 53.977)
  line L409 (-0.8923, 53.977) -> (-1.7756, 53.977)
  line L410 (-1.7756, 53.977) -> (-2.6589, 53.977)
  line L411 (-2.6589, 53.977) -> (-2.6424, 54.6364)
  spline S459 degree 3 poles (-2.6424, 54.6364) (-2.6297, 55.1506) (-2.6114, 55.3291) (-2.5595, 55.4484) knots 0 0 0 0 1 1 1 1
  line L412 (1.955, -37.3629) -> (3.2389, -37.3629)
  line L413 (3.2389, -37.3629) -> (3.2276, -36.0923)
  line L414 (3.2276, -36.0923) -> (3.2162, -34.8214)
  line L415 (3.2162, -34.8214) -> (3.1062, -34.5833)
  spline S460 degree 3 poles (3.1062, -34.5833) (2.6501, -33.5958) (1.267, -33.6189) (0.8037, -34.6219) knots 0 0 0 0 1 1 1 1
  line L416 (0.8037, -34.6219) -> (0.6937, -34.8599)
  line L417 (0.6937, -34.8599) -> (0.6823, -36.1112)
  line L418 (0.6823, -36.1112) -> (0.671, -37.3629)
  line L419 (0.671, -37.3629) -> (1.955, -37.3629)
  line L420 (1.955, 53.3654) -> (3.2389, 53.3654)
  line L421 (3.2389, 53.3654) -> (3.2276, 54.6364)
  line L422 (3.2276, 54.6364) -> (3.2162, 55.9069)
  line L423 (3.2162, 55.9069) -> (3.1062, 56.1453)
  spline S461 degree 3 poles (3.1062, 56.1453) (2.6501, 57.1328) (1.267, 57.1094) (0.8037, 56.1068) knots 0 0 0 0 1 1 1 1
  line L424 (0.8037, 56.1068) -> (0.6937, 55.8687)
  line L425 (0.6937, 55.8687) -> (0.6823, 54.6171)
  line L426 (0.6823, 54.6171) -> (0.671, 53.3654)
  line L427 (0.671, 53.3654) -> (1.955, 53.3654)
  spline S462 degree 3 poles (1.224, -34.9552) (1.4514, -34.5276) (1.913, -34.3677) (2.3336, -34.5713) knots 0 0 0 0 1 1 1 1
  spline S463 degree 3 poles (2.3336, -34.5713) (2.7058, -34.7515) (2.7767, -34.9786) (2.7767, -35.9932) knots 0 0 0 0 1 1 1 1
  line L428 (2.7767, -35.9932) -> (2.7767, -36.7517)
  line L429 (2.7767, -36.7517) -> (1.9519, -36.7517)
  line L430 (1.9519, -36.7517) -> (1.1267, -36.7517)
  line L431 (1.1267, -36.7517) -> (1.1398, -35.9203)
  spline S464 degree 3 poles (1.1398, -35.9203) (1.1511, -35.199) (1.1621, -35.0714) (1.224, -34.9552) knots 0 0 0 0 1 1 1 1
  spline S465 degree 3 poles (1.224, 55.7731) (1.4514, 56.201) (1.913, 56.3606) (2.3336, 56.1573) knots 0 0 0 0 1 1 1 1
  spline S466 degree 3 poles (2.3336, 56.1573) (2.7058, 55.9768) (2.7767, 55.7501) (2.7767, 54.7354) knots 0 0 0 0 1 1 1 1
  line L432 (2.7767, 54.7354) -> (2.7767, 53.977)
  line L433 (2.7767, 53.977) -> (1.9519, 53.977)
  line L434 (1.9519, 53.977) -> (1.1267, 53.977)
  line L435 (1.1267, 53.977) -> (1.1398, 54.8083)
  spline S467 degree 3 poles (1.1398, 54.8083) (1.1511, 55.5293) (1.1621, 55.6572) (1.224, 55.7731) knots 0 0 0 0 1 1 1 1
  spline S468 degree 3 poles (8.4736, 20.7726) (8.6081, 19.748) (9.5217, 18.8551) (10.4352, 18.8551) knots 0 0 0 0 1 1 1 1
  line L436 (10.4352, 18.8551) -> (10.5732, 18.8551)
  line L437 (10.5732, 18.8551) -> (10.5732, 19.5763)
  line L438 (10.5732, 19.5763) -> (10.5732, 20.2973)
  line L439 (10.5732, 20.2973) -> (10.4346, 20.32)
  spline S469 degree 3 poles (10.4346, 20.32) (9.6194, 20.4521) (9.6335, 21.6779) (10.4524, 21.8544) knots 0 0 0 0 1 1 1 1
  spline S470 degree 3 poles (10.4524, 21.8544) (10.8304, 21.9359) (10.7613, 21.9906) (12.5523, 20.1896) knots 0 0 0 0 1 1 1 1
  spline S471 degree 3 poles (12.5523, 20.1896) (13.9175, 18.8169) (14.2019, 18.5486) (14.2896, 18.5489) knots 0 0 0 0 1 1 1 1
  line L440 (14.2896, 18.5489) -> (14.3949, 18.5493)
  line L441 (14.3949, 18.5493) -> (14.3949, 20.9381)
  line L442 (14.3949, 20.9381) -> (14.3949, 23.3265)
  line L443 (14.3949, 23.3265) -> (13.7641, 23.3265)
  line L444 (13.7641, 23.3265) -> (13.1336, 23.3265)
  line L445 (13.1336, 23.3265) -> (13.1336, 22.4776)
  line L446 (13.1336, 22.4776) -> (13.1336, 21.6291)
  line L447 (13.1336, 21.6291) -> (12.5317, 22.2252)
  spline S472 degree 3 poles (12.5317, 22.2252) (11.6546, 23.0937) (11.2728, 23.3038) (10.5732, 23.3028) knots 0 0 0 0 1 1 1 1
  spline S473 degree 3 poles (10.5732, 23.3028) (9.2696, 23.3004) (8.2958, 22.1271) (8.4736, 20.7726) knots 0 0 0 0 1 1 1 1
  spline S474 degree 3 poles (8.475, 26.0139) (8.5933, 24.9882) (9.3232, 24.1524) (10.3211, 23.8999) knots 0 0 0 0 1 1 1 1
  spline S475 degree 3 poles (10.3211, 23.8999) (10.709, 23.8019) (12.2562, 23.7884) (12.6871, 23.8799) knots 0 0 0 0 1 1 1 1
  spline S476 degree 3 poles (12.6871, 23.8799) (15.1898, 24.4103) (15.2255, 28.2534) (12.7339, 28.8866) knots 0 0 0 0 1 1 1 1
  spline S477 degree 3 poles (12.7339, 28.8866) (12.3514, 28.9839) (10.6409, 28.9692) (10.2667, 28.8653) knots 0 0 0 0 1 1 1 1
  spline S478 degree 3 poles (10.2667, 28.8653) (9.0684, 28.5334) (8.3216, 27.345) (8.475, 26.0139) knots 0 0 0 0 1 1 1 1
  spline S479 degree 3 poles (8.4736, 31.5117) (8.6081, 30.487) (9.5217, 29.5941) (10.4352, 29.5941) knots 0 0 0 0 1 1 1 1
  line L448 (10.4352, 29.5941) -> (10.5732, 29.5941)
  line L449 (10.5732, 29.5941) -> (10.5732, 30.3154)
  line L450 (10.5732, 30.3154) -> (10.5732, 31.0363)
  line L451 (10.5732, 31.0363) -> (10.4346, 31.059)
  spline S480 degree 3 poles (10.4346, 31.059) (9.6194, 31.1911) (9.6335, 32.417) (10.4524, 32.5934) knots 0 0 0 0 1 1 1 1
  spline S481 degree 3 poles (10.4524, 32.5934) (10.8304, 32.675) (10.7613, 32.73) (12.5523, 30.9287) knots 0 0 0 0 1 1 1 1
  spline S482 degree 3 poles (12.5523, 30.9287) (13.9175, 29.5559) (14.2019, 29.2877) (14.2896, 29.288) knots 0 0 0 0 1 1 1 1
  line L452 (14.2896, 29.288) -> (14.3949, 29.2883)
  line L453 (14.3949, 29.2883) -> (14.3949, 31.6771)
  line L454 (14.3949, 31.6771) -> (14.3949, 34.0656)
  line L455 (14.3949, 34.0656) -> (13.7641, 34.0656)
  line L456 (13.7641, 34.0656) -> (13.1336, 34.0656)
  line L457 (13.1336, 34.0656) -> (13.1336, 33.217)
  line L458 (13.1336, 33.217) -> (13.1336, 32.3681)
  line L459 (13.1336, 32.3681) -> (12.5317, 32.9642)
  spline S483 degree 3 poles (12.5317, 32.9642) (11.6546, 33.8331) (11.2728, 34.0429) (10.5732, 34.0418) knots 0 0 0 0 1 1 1 1
  spline S484 degree 3 poles (10.5732, 34.0418) (9.2696, 34.0398) (8.2958, 32.8662) (8.4736, 31.5117) knots 0 0 0 0 1 1 1 1
  spline S485 degree 3 poles (8.4716, 36.4028) (8.5947, 35.5766) (9.2692, 34.9145) (10.0283, 34.8746) knots 0 0 0 0 1 1 1 1
  line L460 (10.0283, 34.8746) -> (10.3056, 34.8598)
  line L461 (10.3056, 34.8598) -> (10.3056, 35.5663)
  line L462 (10.3056, 35.5663) -> (10.3056, 36.2724)
  line L463 (10.3056, 36.2724) -> (10.1487, 36.2975)
  spline S486 degree 3 poles (10.1487, 36.2975) (9.7834, 36.356) (9.6514, 36.7058) (9.9004, 36.9548) knots 0 0 0 0 1 1 1 1
  spline S487 degree 3 poles (9.9004, 36.9548) (10.2206, 37.2751) (10.6877, 36.9913) (10.6877, 36.4771) knots 0 0 0 0 1 1 1 1
  line L464 (10.6877, 36.4771) -> (10.6877, 36.2824)
  line L465 (10.6877, 36.2824) -> (11.3564, 36.2824)
  line L466 (11.3564, 36.2824) -> (12.0254, 36.2824)
  line L467 (12.0254, 36.2824) -> (12.0257, 36.5404)
  spline S488 degree 3 poles (12.0257, 36.5404) (12.0261, 37.1302) (12.3184, 37.4587) (12.7676, 37.3745) knots 0 0 0 0 1 1 1 1
  spline S489 degree 3 poles (12.7676, 37.3745) (13.5264, 37.2324) (13.428, 35.9721) (12.6531, 35.9078) knots 0 0 0 0 1 1 1 1
  line L468 (12.6531, 35.9078) -> (12.4457, 35.8906)
  line L469 (12.4457, 35.8906) -> (12.4457, 35.1834)
  line L470 (12.4457, 35.1834) -> (12.4457, 34.4763)
  line L471 (12.4457, 34.4763) -> (12.7147, 34.5028)
  spline S490 degree 3 poles (12.7147, 34.5028) (13.8566, 34.6152) (14.5858, 35.45) (14.5858, 36.6453) knots 0 0 0 0 1 1 1 1
  spline S491 degree 3 poles (14.5858, 36.6453) (14.5858, 38.4906) (12.6861, 39.4702) (11.4358, 38.2698) knots 0 0 0 0 1 1 1 1
  spline S492 degree 3 poles (11.4358, 38.2698) (11.2215, 38.0638) (11.1899, 38.0452) (11.1445, 38.0999) knots 0 0 0 0 1 1 1 1
  spline S493 degree 3 poles (11.1445, 38.0999) (10.8088, 38.5044) (9.9864, 38.6564) (9.4539, 38.4122) knots 0 0 0 0 1 1 1 1
  spline S494 degree 3 poles (9.4539, 38.4122) (8.7681, 38.0978) (8.3471, 37.2369) (8.4716, 36.4028) knots 0 0 0 0 1 1 1 1
  spline S495 degree 3 poles (8.8609, 21.6642) (9.1911, 22.6782) (10.383, 23.2003) (11.3154, 22.7394) knots 0 0 0 0 1 1 1 1
  spline S496 degree 3 poles (11.3154, 22.7394) (11.5789, 22.609) (11.712, 22.4969) (12.4391, 21.7935) knots 0 0 0 0 1 1 1 1
  spline S497 degree 3 poles (12.4391, 21.7935) (13.0246, 21.2273) (13.2898, 20.9952) (13.352, 20.9952) knots 0 0 0 0 1 1 1 1
  line L472 (13.352, 20.9952) -> (13.4394, 20.9952)
  line L473 (13.4394, 20.9952) -> (13.4394, 21.9507)
  line L474 (13.4394, 21.9507) -> (13.4394, 22.9062)
  line L475 (13.4394, 22.9062) -> (13.7641, 22.9062)
  line L476 (13.7641, 22.9062) -> (14.0891, 22.9062)
  line L477 (14.0891, 22.9062) -> (14.0888, 21.043)
  line L478 (14.0888, 21.043) -> (14.0888, 19.1801)